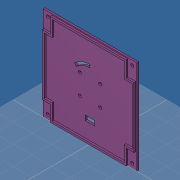
# Autodesk Inventor part: DayLightGlow_BaseCover
Saved by Autodesk Inventor 2019 (Build 230136000, 136)
## iProperties
Created: 2019-01-03
Part Number: DayLightGlow_BaseCover
Material: Generisch
Document SubType Name: Modeling
Designer: Stefan
Mass: 20.2009 g
Surface Area: 212.922 cm^2
Volume: 20.2009 cm^3
Density: 1 g/cm^3
Appearance: Glatt - Violett
Author: Stefan
Autodesk Inventor part; units mm, degrees
ref_plane "YZ Plane" through (0, 0, 0) normal (1, 0, 0) x (0, 1, 0)
ref_plane "XZ Plane" through (0, 0, 0) normal (0, 1, 0) x (-1, 0, 0)
ref_plane "XY Plane" through (0, 0, 0) normal (0, 0, 1) x (1, 0, 0)
sketch "Skizze1" plane through (0, 0, 0) normal (0, 0, 1) x (1, 0, 0)
  line L0 (48.8, -48.8) -> (-48.8, -48.8)
  line L1 (-48.8, -48.8) -> (-48.8, 48.8)
  line L2 (-48.8, 48.8) -> (48.8, 48.8)
  line L3 (48.8, 48.8) -> (48.8, -48.8)
  line L4 (48.8, -48.8) -> (-48.8, 48.8) construction
  line L5 (-48.8, -48.8) -> (48.8, 48.8) construction
  line L6 (-50, 50) -> (50, 50) construction
  line L7 (50, 50) -> (50, -50) construction
  line L8 (50, -50) -> (-50, -50) construction
  line L9 (-50, -50) -> (-50, 50) construction
  line L10 (-50, 50) -> (50, -50) construction
  line L11 (50, 50) -> (-50, -50) construction
  line L12 (47.75, -47.75) -> (-47.75, -47.75)
  line L13 (-47.75, -47.75) -> (-47.75, 47.75)
  line L14 (-47.75, 47.75) -> (47.75, 47.75)
  line L15 (47.75, 47.75) -> (47.75, -47.75)
  line L16 (47.75, -47.75) -> (-47.75, 47.75) construction
  line L17 (-47.75, -47.75) -> (47.75, 47.75) construction
  circle A0 centre (0, 0) radius 15 construction
  line L18 (-50, 50) -> (-39.5, 50) construction
  line L19 (-39.5, 50) -> (-39.5, 31.5) construction
  line L20 (-39.5, 31.5) -> (-50, 31.5) construction
  line L21 (-50, 31.5) -> (-50, 50) construction
  line L22 (50, 50) -> (39.5, 50) construction
  line L23 (39.5, 50) -> (39.5, 31.5) construction
  line L24 (39.5, 31.5) -> (50, 31.5) construction
  line L25 (50, 31.5) -> (50, 50) construction
  line L26 (-50, -50) -> (-39.5, -50) construction
  line L27 (-39.5, -50) -> (-39.5, -31.5) construction
  line L28 (-39.5, -31.5) -> (-50, -31.5) construction
  line L29 (-50, -31.5) -> (-50, -50) construction
  line L30 (50, -50) -> (39.5, -50) construction
  line L31 (39.5, -50) -> (39.5, -31.5) construction
  line L32 (39.5, -31.5) -> (50, -31.5) construction
  line L33 (50, -31.5) -> (50, -50) construction
  line L34 (-39.5, 47.75) -> (39.5, 47.75)
  line L35 (39.5, 47.75) -> (39.5, 45.75)
  line L36 (39.5, 45.75) -> (-39.5, 45.75)
  line L37 (-39.5, 45.75) -> (-39.5, 47.75)
  line L38 (47.75, 31.5) -> (45.75, 31.5)
  line L39 (45.75, 31.5) -> (45.75, -31.5)
  line L40 (45.75, -31.5) -> (47.75, -31.5)
  line L41 (47.75, -31.5) -> (47.75, 31.5)
  line L42 (39.5, -47.75) -> (-39.5, -47.75)
  line L43 (-39.5, -47.75) -> (-39.5, -45.75)
  line L44 (-39.5, -45.75) -> (39.5, -45.75)
  line L45 (39.5, -45.75) -> (39.5, -47.75)
  line L46 (-47.75, -31.5) -> (-45.75, -31.5)
  line L47 (-45.75, -31.5) -> (-45.75, 31.5)
  line L48 (-45.75, 31.5) -> (-47.75, 31.5)
  line L49 (-47.75, 31.5) -> (-47.75, -31.5)
  line L50 (-39.5, 45.75) -> (-39.5, 31.5)
  line L51 (-45.75, 31.5) -> (-39.5, 31.5)
  line L52 (39.5, 45.75) -> (39.5, 31.5)
  line L53 (39.5, 31.5) -> (45.75, 31.5)
  line L54 (45.75, -31.5) -> (39.5, -31.5)
  line L55 (39.5, -31.5) -> (39.5, -45.75)
  line L56 (-39.5, -45.75) -> (-39.5, -31.5)
  line L57 (-45.75, -31.5) -> (-39.5, -31.5)
  line L58 (-45.75, -29.5) -> (-37.5, -29.5)
  line L59 (-37.5, -29.5) -> (-37.5, -45.75)
  line L60 (45.75, -29.5) -> (37.5, -29.5)
  line L61 (37.5, -29.5) -> (37.5, -45.75)
  line L62 (37.5, 45.75) -> (37.5, 29.5)
  line L63 (37.5, 29.5) -> (45.75, 29.5)
  line L64 (-37.5, 45.75) -> (-37.5, 29.5)
  line L65 (-37.5, 29.5) -> (-45.75, 29.5)
  line L66 (-39.5, 45.75) -> (-37.5, 45.75)
  line L67 (-45.75, 29.5) -> (-45.75, 31.5)
  line L68 (37.5, 45.75) -> (39.5, 45.75)
  line L69 (45.75, 29.5) -> (45.75, 31.5)
  line L70 (45.75, -29.5) -> (45.75, -31.5)
  line L71 (37.5, -45.75) -> (39.5, -45.75)
  line L72 (-39.5, -45.75) -> (-37.5, -45.75)
  line L73 (-45.75, -31.5) -> (-45.75, -29.5)
  point P0 (0, 0)
  point P1 (0, 0)
  point P2 (-10.6066, 10.6066)
  point P3 (10.6066, 10.6066)
  point P4 (10.6066, -10.6066)
  point P5 (-10.6066, -10.6066)
  point P6 (-44, 44)
  point P7 (44, 44)
  point P8 (44, -44)
  point P9 (-44, -44)
  dimension "d0" = 97.6
  dimension "d55" = 30
  dimension "d61" = 100
  dimension "d62" = 95.5
  dimension "d63" = 18.5
  dimension "d64" = 10.5
  dimension "d65" = 2
  dimension "d67" = 6
  constraints: 148 end point, 29 point on line, 23 parallel, 19 perpendicular, 15 equal length, 14 collinear, 13 horizontal, 12 midpoint, 4 point on circle, 3 vertical, 2 vertical alignment, 1 centre point, 1 coincident, 1 horizontal alignment
  measures "d0" distance of L0.end L1.end
  measures "d55" diameter of A0
  measures "d61" distance of L6.end L7.end
  measures "d62" distance of L13.end L14.end
  measures "d63" distance between parallel lines of L20 L18
  measures "d64" distance between parallel lines of L19 L21
  measures "d65" distance between parallel lines of L36 L34
  measures "d67" distance from line of point (-44, 44) L9
extrude "Extrusion1" add sketch "Skizze1" against normal blind 2 contours L0 L1 L2 L3 | L12 L45 L55 L54 L40 L15 | L12 L43 L44 L45 | L40 L39 L38 L15 | L12 L13 L46 L57 L56 L43 | L44 L61 L60 L39 L54 L55 | L38 L53 L52 L35 L14 L15 | L56 L57 L47 L58 L59 L44 | L44 L59 L58 L47 L65 L64 L36 L62 L63 L39 L60 L61 | L39 L63 L62 L36 L52 L53 | L13 L48 L47 L46 | L35 L36 L37 L14 | L13 L14 L37 L50 L51 L48 | L51 L50 L36 L64 L65 L47
hole "Bohrung1" at (-10.6066, 10.6066, 0) at (10.6066, 10.6066, 0) at (-10.6066, -10.6066, 0) at (10.6066, -10.6066, 0) at (-44, 44, 0) at (44, 44, 0) at (44, -44, 0) at (-44, -44, 0) direction (0, 0, -1) diameter 3.4 end through all
extrude "Extrusion4" add sketch "Skizze1" along normal blind 2 contours L12 L43 L44 L45 | L40 L39 L38 L15 | L44 L61 L60 L39 L54 L55 | L56 L57 L47 L58 L59 L44 | L39 L63 L62 L36 L52 L53 | L13 L48 L47 L46 | L35 L36 L37 L14 | L51 L50 L36 L64 L65 L47
sketch "Skizze2" plane through (0, 0, -2) normal (0, 0, -1) x (-1, 0, 0)
  line L0 (-50, -50) -> (50, -50) construction
  line L1 (50, -50) -> (50, 50) construction
  line L2 (50, 50) -> (-50, 50) construction
  line L3 (-50, 50) -> (-50, -50) construction
  line L4 (-50, -50) -> (50, 50) construction
  line L5 (50, -50) -> (-50, 50) construction
  circle A0 centre (0, 0) radius 20 construction
  line L6 (0, 20) -> (0, 23)
  arc A1 (14.1421, 14.1421) -> (0, 20) centre (0, 0) ccw
  arc A2 (16.2635, 16.2635) -> (0, 23) centre (0, 0) ccw
  line L7 (14.1421, 14.1421) -> (16.2635, 16.2635)
  line L8 (-5, -25) -> (5, -25)
  line L9 (5, -25) -> (5, -30)
  line L10 (5, -30) -> (-5, -30)
  line L11 (-5, -30) -> (-5, -25)
  line L12 (-5, -25) -> (5, -30) construction
  line L13 (5, -25) -> (-5, -30) construction
  point P0 (0, 0)
  point P1 (0, 0)
  point P2 (0, -27.5)
  point P3 (0, -27.5)
  dimension "d45" = 100
  dimension "d46" = 100
  dimension "d47" = 40
  dimension "d53" = 3
  dimension "d54" = 45
  dimension "d57" = 10
  dimension "d58" = 5
  dimension "d59" = 25
  constraints: 28 end point, 7 midpoint, 6 point on circle, 4 parallel, 3 centre point, 3 concentric, 2 horizontal, 2 perpendicular, 2 vertical alignment, 1 coincident, 1 line through centre, 1 vertical
  measures "d45" distance of L1.end L2.end
  measures "d46" distance of L2.end L0.start
  measures "d47" diameter of A0
  measures "d53" radial gap between concentric circles of A0 A2
  measures "d54" angle of L7 L6
  measures "d57" distance between parallel lines of L9 L11
  measures "d58" distance between parallel lines of L10 L8
  measures "d59" distance from line of point (0, 0) L8
extrude "Extrusion5" cut sketch "Skizze2" against normal through all
